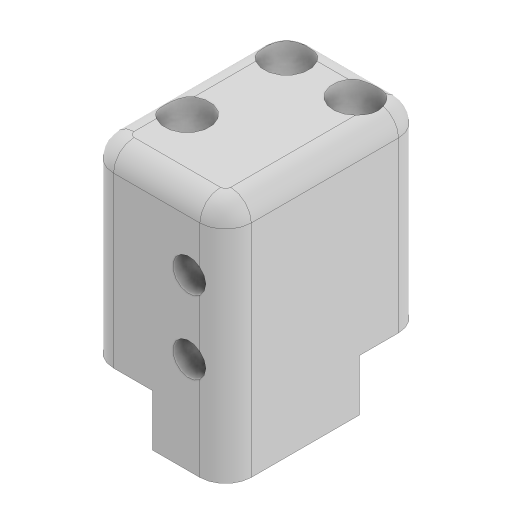
# Autodesk Inventor part: left foot link
Saved by Autodesk Inventor 2024 (Build 280153000, 153)
## iProperties
Created: 2023-09-29
Part Number: left foot link
Material: Generic
Document SubType Name: Modeling
Designer: chris
Density: 1 g/cm^3
Appearance: Default
Author: chris
Autodesk Inventor part; units mm, degrees
ref_plane "YZ Plane" through (0, 0, 0) normal (1, 0, 0) x (0, 1, 0)
ref_plane "XZ Plane" through (0, 0, 0) normal (0, 1, 0) x (-1, 0, 0)
sketch "Sketch1" plane through (0, 0, 0) normal (0, 0, 1) x (1, 0, 0)
  line L0 (0, 29.725) -> (0, 0)
  line L1 (9, 0) -> (0, 0)
  circle A0 centre (4.5, 11.95) radius 2
  circle A1 centre (4.5, 20.95) radius 2
  line L2 (0, 29.725) -> (9, 29.725)
  line L3 (9, 29.725) -> (9, 0)
  constraints: 8 end point, 2 centre point, 1 horizontal, 1 perpendicular
extrude "Extrusion1" add sketch "Sketch1" along normal blind 16.51
sketch "Sketch2" plane through (0, 29.725, 0) normal (0, 1, 0) x (1, 0, 0)
  circle A0 centre (4.5, 4) radius 1.5
  circle A1 centre (13, 4) radius 1.5
  circle A2 centre (13, -8.255) radius 1.5
  arc A3 (3.175, 8) -> (0, 4.825) centre (3.175, 4.825) ccw
  line L0 (0, 4.825) -> (0, 0)
  line L1 (9, 0) -> (0, 0)
  line L2 (9, -16.51) -> (9, 0)
  line L3 (9, -16.51) -> (13.825, -16.51)
  arc A4 (13.825, -16.51) -> (17, -13.335) centre (13.825, -13.335) ccw
  line L4 (17, -13.335) -> (17, 4.825)
  arc A5 (17, 4.825) -> (13.825, 8) centre (13.825, 4.825) ccw
  line L5 (13.825, 8) -> (3.175, 8)
  line L6 (9, 0) -> (0, 0) projected
  line L7 (0, 0) -> (0, -16.51) projected
  line L8 (9, -16.51) -> (0, -16.51) projected
  line L9 (9, 0) -> (9, -16.51) projected
  constraints: 12 end point, 6 centre point, 6 point on circle
extrude "Extrusion2" add sketch "Sketch2" against normal blind 23.368 contours L5 A5 L4 A4 L3 L2 L1 L0 A3
fillet "Fillet1" radius 3.175 1 edges at (0, 14.8625, 16.51)
fillet "Fillet2" radius 2.54 8 edges at (0.9299, 29.725, 15.5801) (8.5, 29.725, 16.51) (16.0701, 29.725, 15.5801) (17, 29.725, 4.255) (16.0701, 29.725, -7.0701) (8.5, 29.725, -8) (0.9299, 29.725, -7.0701) (0, 29.725, 4.255)
sketch "Sketch3" plane through (4.5, 29.725, -4) normal (0, 1, 0) x (1, 0, 0)
  circle A0 centre (0, 0) radius 1.5 projected
  circle A1 centre (0, 0) radius 2.75
  circle A2 centre (8.5, 0) radius 1.5 projected
  circle A3 centre (8.5, 0) radius 2.75
  circle A4 centre (8.5, -12.255) radius 1.5 projected
  circle A5 centre (8.5, -12.255) radius 2.75
  point P0 (-4.5, -4)
  dimension "d6" = 5.5
  dimension "d7" = 5.5
  dimension "d8" = 5.5
  constraints: 3 centre point, 3 coincident
  measures "d6" diameter of A1
  measures "d7" diameter of A3
  measures "d8" diameter of A5
extrude "Extrusion3" cut sketch "Sketch3" against normal blind 15.875
sketch "Sketch4" plane through (3.175, 29.725, 13.97) normal (0, 1, 0) x (1, 0, 0)
  line L0 (-3.175, 13.97) -> (-3.175, 0.635) projected
  line L1 (-3.175, 13.97) -> (-34.3982, 13.97)
  line L2 (-34.3982, 13.97) -> (-34.3982, 35.7562)
  line L3 (-34.3982, 35.7562) -> (-34.3982, -7.8899)
  constraints: 6 end point, 1 horizontal, 1 perpendicular, 1 point on line
sketch "Sketch5" plane through (0, 0, 16.51) normal (0, 0, 1) x (1, 0, 0)
  line L0 (-31.2232, 29.725) -> (-31.2232, 10.8959)
  point P0 (0, 0)
  constraints: 2 end point, 1 vertical
ref_plane "Work Plane1" through (-31.2232, 29.725, -21.7862) normal (1, 0, 0) x (0, 0, 1)
mirror "Mirror1" about plane through (-31.2232, 29.725, -21.7862) normal (1, 0, 0) of "Extrusion1", "Extrusion2", "Fillet1", "Fillet2", "Extrusion3"
sketch "Sketch6" plane through (3.175, 29.725, 13.97) normal (0, 1, 0) x (1, 0, 0)
  line L0 (-3.175, 30.7572) -> (31.9746, 31.4773)
  line L1 (31.9746, 31.4773) -> (32.7916, -8.3997)
  line L2 (32.7916, -8.3997) -> (-13.1213, -13.2586)
  line L3 (-13.1213, -13.2586) -> (-3.175, 30.7572)
  point P0 (-3.175, 13.97)
  constraints: 8 end point, 1 perpendicular
extrude "Extrusion4" cut sketch "Sketch6" against normal through all
body "Solid1"
